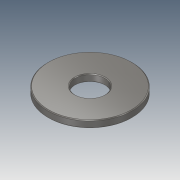
# Autodesk Inventor part: 900-80-WASHERS-DIN9021-M8
Saved by Autodesk Inventor 2018.2 (Build 222227000, 227)
## iProperties
Manager: feesmrt
Company: FRANCOR
Part Number: 900-80-WASHERS-DIN9021-M8
Project: Rescue Robot
Cost Center: -
Material: Edelstahl
Description: Unterlegscheibe DIN 9021 - M8
Document SubType Name: Modeling
Designer: feesmrt
Engineer: feesmrt
Authority: feesmrt
Density: 8 g/cm^3
Appearance: Halbpoliert
Stock Number: 900-80-WASHERS-DIN9021-M8
Title: Unterlegscheibe DIN 9021 - M8
Subject: Rescue Robot
Author: feesmrt
Revision Number: 1
Autodesk Inventor part; units mm, degrees
ref_plane "YZ Plane" through (0, 0, 0) normal (1, 0, 0) x (0, 1, 0)
ref_plane "XZ Plane" through (0, 0, 0) normal (0, 1, 0) x (-1, 0, 0)
ref_plane "XY Plane" through (0, 0, 0) normal (0, 0, 1) x (1, 0, 0)
sketch "Skizze1" plane through (0, 0, 0) normal (0, 0, 1) x (1, 0, 0)
  circle A0 centre (0, 0) radius 4.2
  circle A1 centre (0, 0) radius 12
  dimension "d0" = 24
  dimension "d1" = 8.4
  constraints: 2 centre point, 2 coincident
  measures "d0" diameter of A1
  measures "d1" diameter of A0
extrude "Extrusion1" add sketch "Skizze1" along normal mid plane 2
chamfer "Fase1" distance 0.2 angle 45 4 edges at (-12, 0, 1) (-12, 0, -1) (-4.2, 0, 1) (-4.2, 0, -1)
